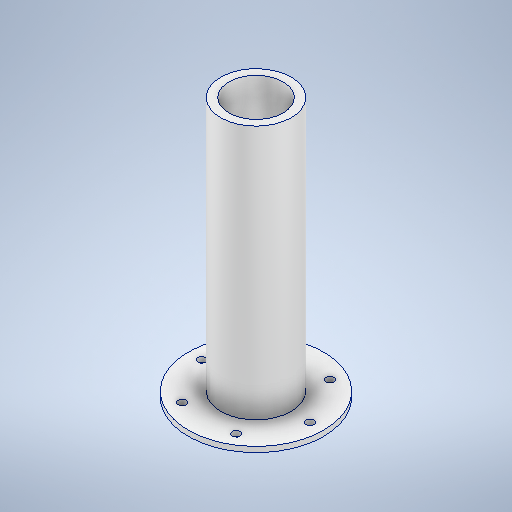
# Autodesk Inventor part: CylinderAttachment
Saved by Autodesk Inventor 2025.2 (Build 292293000, 293)
## iProperties
Created: 2025-07-17
Part Number: CylinderAttachment
Material: Generic
Document SubType Name: Modeling
Designer: Simon
Density: 1 g/cm^3
Appearance: Aluminum - Flat
Author: Simon
Autodesk Inventor part; units mm, degrees
ref_plane "YZ Plane" through (0, 0, 0) normal (1, 0, 0) x (0, 1, 0)
ref_plane "XZ Plane" through (0, 0, 0) normal (0, 1, 0) x (-1, 0, 0)
ref_plane "XY Plane" through (0, 0, 0) normal (0, 0, 1) x (1, 0, 0)
sketch "Sketch1" plane through (0, 0, 0) normal (0, 1, 0) x (-1, 0, 0)
  circle A0 centre (0, 0) radius 3
  dimension "d0" = 6
  constraints: 1 centre point, 1 coincident
  measures "d0" diameter of A0
extrude "Extrusion1" add sketch "Sketch1" along normal blind 5.5
sketch "Sketch2" plane through (0, 5.5, 0) normal (0, 1, 0) x (1, 0, 0)
  circle A0 centre (0, 0) radius 25
  dimension "d3" = 50
  constraints: 1 centre point, 1 coincident
  measures "d3" diameter of A0
extrude "Extrusion2" add sketch "Sketch2" along normal blind 2
sketch "Sketch3" plane through (0, 7.5, 0) normal (0, 1, 0) x (1, 0, 0)
  circle A0 centre (0, 0) radius 13
  circle A1 centre (0, 0) radius 10
  dimension "d6" = 20
  dimension "d24" = 26
  constraints: 2 centre point, 2 coincident
  measures "d6" diameter of A1
  measures "d24" diameter of A0
extrude "Extrusion3" add sketch "Sketch3" along normal blind 94
sketch "Sketch4" plane through (0, 0, 0) normal (0, -1, 0) x (1, 0, 0)
  circle A0 centre (0, 0) radius 1
  dimension "d9" = 2
  constraints: 1 centre point, 1 coincident
  measures "d9" diameter of A0
extrude "Extrusion4" cut sketch "Sketch4" against normal through all
thread "Thread2" size "M6x1" class "6g" standard "ANSI Metric M Profile" full length
sketch "Sketch5" plane through (0, 7.5, 0) normal (0, 1, 0) x (1, 0, 0)
  circle A0 centre (0, 0) radius 1 projected
  circle A1 centre (0, 0) radius 20
  circle A2 centre (-20, 0) radius 1.5
  circle A3 centre (-10, -17.3205) radius 1.5
  circle A4 centre (10, -17.3205) radius 1.5
  circle A5 centre (20, 0) radius 1.5
  circle A6 centre (10, 17.3205) radius 1.5
  circle A7 centre (-10, 17.3205) radius 1.5
  dimension "d16" = 40
  dimension "d17" = 3
  dimension "d20" = 360
  constraints: 6 centre point, 1 coincident, 1 horizontal alignment, 15 other
  measures "d17" diameter of A2
extrude "Extrusion5" cut sketch "Sketch5" against normal through all contours A1 A5 | A1 A5 | A6 A1 | A1 A6 | A4 A1 | A1 A4 | A7 A1 | A1 A7 | A3 A1 | A1 A3 | A2 A1 | A1 A2
body "Solid1"
